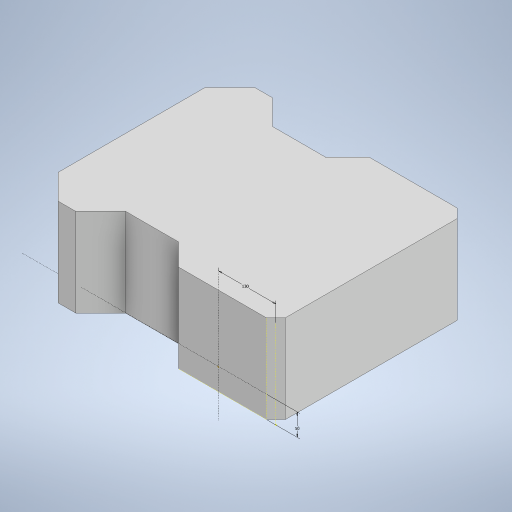
# Autodesk Inventor part: Frame
Saved by Autodesk Inventor 2024 (Build 280153000, 153)
## iProperties
Created: 2025-02-27
Part Number: Frame
Material: Generic
Document SubType Name: Modeling
Designer: xehon
Density: 1 g/cm^3
Appearance: Default
Author: xehon
Autodesk Inventor part; units mm, degrees
ref_plane "YZ Plane" through (0, 0, 0) normal (1, 0, 0) x (0, 1, 0)
ref_plane "XZ Plane" through (0, 0, 0) normal (0, 1, 0) x (-1, 0, 0)
ref_plane "XY Plane" through (0, 0, 0) normal (0, 0, 1) x (1, 0, 0)
sketch "Sketch1" plane through (0, 0, 0) normal (0, 1, 0) x (-1, 0, 0)
  line L0 (0.0381, -21.3061) -> (0.0381, -411.3061)
  line L1 (0.0381, -411.3061) -> (21.2513, -432.5193)
  line L2 (0.0381, -411.3061) -> (30.0381, -411.3061) construction
  line L3 (21.2513, -432.5193) -> (221.2513, -432.5193)
  line L4 (221.2513, -432.5193) -> (270.7487, -383.0218)
  line L5 (270.7487, -383.0218) -> (390.7487, -383.0218)
  line L6 (390.7487, -383.0218) -> (447.3173, -439.5904)
  line L7 (447.3173, -439.5904) -> (487.3173, -439.5904)
  line L8 (487.3173, -439.5904) -> (543.8858, -383.0218)
  line L9 (-53.2718, -216.3061) -> (592.6367, -216.3061) construction
  line L10 (0.0381, -21.3061) -> (21.2513, -0.0929)
  line L11 (21.2513, -0.0929) -> (221.2513, -0.0929)
  line L12 (221.2513, -0.0929) -> (270.7487, -49.5904)
  line L13 (270.7487, -49.5904) -> (390.7487, -49.5904)
  line L14 (390.7487, -49.5904) -> (447.3173, 6.9782)
  line L15 (447.3173, 6.9782) -> (487.3173, 6.9782)
  line L16 (487.3173, 6.9782) -> (543.8858, -49.5904)
  line L17 (543.8858, -383.0218) -> (543.8858, -49.5904)
  point P0 (0, 0)
  dimension "d0" = 390
  dimension "d1" = 30
  dimension "d2" = 45
  dimension "d3" = 70
  dimension "d4" = 135
  dimension "d5" = 200
  dimension "d6" = 120
  dimension "d7" = 80
  dimension "d8" = 135
  dimension "d9" = 226.066
  dimension "d10" = 21.2132
  dimension "d11" = 40
  dimension "d12" = 80
  dimension "d15" = 543.8478
  constraints: 36 end point, 7 symmetric about line, 5 horizontal, 2 vertical, 1 equal length, 1 perpendicular
  measures "d0" distance of L0.start L0.end
  measures "d1" distance of L0.end L1.end
  measures "d2" angle of L1 L2
  measures "d3" distance of L3.end L4.end
  measures "d4" angle of L4 L3
  measures "d5" distance of L1.end L3.end
  measures "d6" distance of L4.end L5.end
  measures "d7" distance of L5.end L6.end
  measures "d8" angle of L5 L6
  measures "d9" horizontal distance of L6.end L3.end
  measures "d10" horizontal distance of L1.end L0.end
  measures "d11" distance of L6.end L7.end
  measures "d12" distance of L7.end L8.end
  measures "d15" horizontal distance of L0.end L8.end
extrude "Extrusion1" add sketch "Sketch1" along normal blind 200
sketch "Sketch2" plane through (-221.2513, 0, -0.0929) normal (0, 0, 1) x (1, 0, 0)
  line L0 (200, 0) -> (200, 200) construction
  line L1 (200, 50) -> (-356.3945, 50) construction
  line L2 (0, 0) -> (200, 0) construction
  line L3 (91.2132, 236.2215) -> (91.2132, -57.6692) construction
  line L4 (221.2132, 0) -> (221.2132, 200) construction
  point P0 (221.2513, 0)
  dimension "d18" = 50
  dimension "d19" = 130
  constraints: 4 end point, 1 perpendicular, 1 point on line, 1 vertical
  measures "d18" distance between parallel lines of L1 L2
  measures "d19" distance between parallel lines of L4 L3
body "Solid1"
